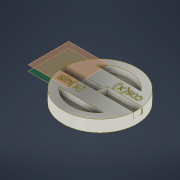
# Autodesk Inventor part: sincos stand
Saved by Autodesk Inventor 2022 (Build 260153000, 153)
## iProperties
Created: 2021-06-07
Part Number: sincos stand
Material: Generic
Document SubType Name: Modeling
Designer: sidsa
Density: 1 g/cm^3
Appearance: Silver
Author: sidsa
## iProperties of the stored document sincos stand_3DPrint.ipt
Created: 2021-06-07
Part Number: sincos stand_3DPrint
Material: Generic
Document SubType Name: Modeling
Designer: sidsa
Density: 1 g/cm^3
Appearance: Default
Author: sidsa
Autodesk Inventor part; units mm, degrees
ref_plane "YZ Plane" through (0, 0, 0) normal (1, 0, 0) x (0, 1, 0)
ref_plane "XZ Plane" through (0, 0, 0) normal (0, 1, 0) x (-1, 0, 0)
ref_plane "XY Plane" through (0, 0, 0) normal (0, 0, 1) x (1, 0, 0)
sketch "Sketch1" plane through (0, 0, 0) normal (0, 1, 0) x (-1, 0, 0)
  line L0 (0, 0) -> (0, 4.7625) construction
  line L1 (-39.8982, 4.7625) -> (0, 4.7625) construction
  line L2 (-39.8982, 0) -> (-39.8982, 4.7625) construction
  line L3 (-39.8982, 0) -> (-19.9491, 0) construction
  line L4 (-19.9491, 0) -> (-19.9491, 3.175) construction
  line L5 (-19.9491, 3.175) -> (-16.0334, 3.175) construction
  line L6 (-19.9491, 0.5949) -> (0, 0.5949) construction
  line L7 (-19.9491, 3.7699) -> (0, 3.7699) construction
  line L8 (-19.9491, 0.5949) -> (-19.9491, 3.7699) construction
  line L9 (-39.8982, 0) -> (-20.8482, 0)
  line L10 (-20.8482, 0) -> (-20.8482, 4.7625)
  line L11 (-20.8482, 4.7625) -> (-39.8982, 4.7625)
  line L12 (-39.8982, 4.7625) -> (-39.8982, 0)
  circle A0 centre (-19.9491, 2.9762) radius 20.0907
  line L13 (0, 4.7625) -> (-19.9491, 4.7625)
  line L14 (-19.9491, 4.7625) -> (-19.9491, 1.5875)
  line L15 (-19.9491, 1.5875) -> (0, 1.5875)
  line L16 (0, 1.5875) -> (0, 4.7625)
  point P0 (-18.8793, 0.5949)
  point P1 (0, 0.5949)
  point P2 (-39.8182, 0)
  point P3 (-39.8982, 0.5949)
  dimension "d1" = 19.05
  dimension "d15" = 3.175
  constraints: 34 end point, 4 parallel, 4 point on line, 2 horizontal, 2 perpendicular, 3 other
  measures "d1" distance of L11.end L10.end
  measures "d15" distance of L13.end L14.end
extrude "Extrusion5" add sketch "Sketch1" along normal blind 3.175 contours L9 L10 L11 L12 A0 picked at (-7.0697, -0.9692)
ref_plane "Work Plane2" through (0, 0, 0) normal (0, -1, 0) x (1, 0, 0)
sketch "Sketch2" plane through (0, 0, 0) normal (0, -1, 0) x (1, 0, 0)
  circle A0 centre (19.9491, 2.9762) radius 20.0907 projected
  circle A1 centre (19.9491, 2.9762) radius 20.0907
  point P0 (0, 0)
  point P1 (39.8982, 0)
  point P2 (39.8199, 0.0117)
  point P3 (40.0398, 2.9762)
  constraints: 1 centre point, 1 coincident, 1 other
extrude "Extrusion2" add sketch "Sketch2" along normal blind 3.175
ref_plane "Work Plane3" through (0, 3.175, 0) normal (0, 1, 0) x (1, 0, 0)
ref_plane "Work Plane1" through (0, 3.175, 0) normal (0, 1, 0) x (1, 0, 0)
sketch "Sketch4" plane through (0, 3.175, 0) normal (0, 1, 0) x (1, 0, 0)
  circle A0 centre (19.9491, -2.9762) radius 20.0907 projected
  circle A1 centre (19.9491, -2.9762) radius 20.0289
  circle A2 centre (19.9491, -2.9762) radius 15.875
  line L0 (32.1471, 7.1838) -> (7.7512, 7.1838)
  line L1 (7.7512, -13.1362) -> (32.1471, -13.1362)
  point P0 (0, 0)
  point P1 (39.8982, -4.7625)
  dimension "d9" = 31.75
  dimension "d10" = 10.16
  dimension "d11" = 10.16
  constraints: 4 end point, 4 point on circle, 2 coincident, 1 centre point, 1 horizontal, 1 parallel, 4 other
  measures "d9" diameter of A2
  measures "d10" distance from line of A2.centre L0
  measures "d11" distance from line of A2.centre L1
extrude "Extrusion4" cut sketch "Sketch4" against normal blind 3.175 contours L0 A2 | A2 L1
sketch "Sketch3" plane through (0, 3.175, 0) normal (0, 1, 0) x (1, 0, 0)
  line L0 (2.8498, -5.5048) -> (33.0797, -5.5048) construction
  line L1 (33.0797, -5.5048) -> (33.0797, -13.0442) construction
  line L2 (33.0797, -13.0442) -> (2.8498, -13.0442) construction
  line L3 (2.8498, -13.0442) -> (2.8498, -5.5048) construction
  line L4 (36.2628, 0.6402) -> (6.0329, 0.6402) construction
  line L5 (6.0329, 0.6402) -> (6.0329, 10.1631) construction
  line L6 (6.0329, 10.1631) -> (36.2628, 10.1631) construction
  line L7 (36.2628, 10.1631) -> (36.2628, 0.6402) construction
  spline S0 degree 2 poles (34.7777, 4.6848) (35.0741, 4.6848) (35.565, 4.5027) (35.741, 4.3174) knots 0 0 0 1 2 2 2
  spline S1 degree 2 poles (35.741, 4.3174) (35.917, 4.1353) (36.1115, 3.5733) (36.1115, 3.1967) knots 0 0 0 1 2 2 2
  spline S2 degree 2 poles (36.1115, 3.1967) (36.1115, 2.82) (35.9108, 2.2704) (35.741, 2.0851) knots 0 0 0 1 2 2 2
  spline S3 degree 2 poles (35.741, 2.0851) (35.5712, 1.8968) (35.0679, 1.6961) (34.7777, 1.6961) knots 0 0 0 1 2 2 2
  spline S4 degree 2 poles (34.7777, 1.6961) (34.543, 1.6961) (34.1046, 1.8289) (33.9348, 1.9153) knots 0 0 0 1 2 2 2
  line L8 (33.9348, 1.9153) -> (33.9348, 2.4556)
  line L9 (33.9348, 2.4556) -> (33.9626, 2.4556)
  spline S5 degree 2 poles (33.9626, 2.4556) (34.0151, 2.4124) (34.1756, 2.3013) (34.2898, 2.2426) knots 0 0 0 1 2 2 2
  spline S6 degree 2 poles (34.2898, 2.2426) (34.3917, 2.1932) (34.6634, 2.116) (34.7869, 2.116) knots 0 0 0 1 2 2 2
  spline S7 degree 2 poles (34.7869, 2.116) (35.1605, 2.116) (35.6144, 2.681) (35.6144, 3.1967) knots 0 0 0 1 2 2 2
  spline S8 degree 2 poles (35.6144, 3.1967) (35.6144, 3.6999) (35.176, 4.2649) (34.7869, 4.2649) knots 0 0 0 1 2 2 2
  spline S9 degree 2 poles (34.7869, 4.2649) (34.5523, 4.2649) (34.1262, 4.0704) (33.9626, 3.9191) knots 0 0 0 1 2 2 2
  line L10 (33.9626, 3.9191) -> (33.9348, 3.9191)
  line L11 (33.9348, 3.9191) -> (33.9348, 4.4594)
  spline S10 degree 2 poles (33.9348, 4.4594) (34.0058, 4.4934) (34.2219, 4.5891) (34.3084, 4.6107) knots 0 0 0 1 2 2 2
  spline S11 degree 2 poles (34.3084, 4.6107) (34.4319, 4.6478) (34.6264, 4.6848) (34.7777, 4.6848) knots 0 0 0 1 2 2 2
  spline S12 degree 2 poles (31.1468, 3.1905) (31.1468, 3.913) (31.8414, 4.7003) (32.4219, 4.7003) knots 0 0 0 1 2 2 2
  spline S13 degree 2 poles (32.4219, 4.7003) (33.0178, 4.7003) (33.7001, 3.8883) (33.7001, 3.1905) knots 0 0 0 1 2 2 2
  spline S14 degree 2 poles (33.7001, 3.1905) (33.7001, 2.4742) (32.9962, 1.6807) (32.4219, 1.6807) knots 0 0 0 1 2 2 2
  spline S15 degree 2 poles (32.4219, 1.6807) (31.8414, 1.6807) (31.1468, 2.4711) (31.1468, 3.1905) knots 0 0 0 1 2 2 2
  spline S16 degree 2 poles (31.6438, 3.1905) (31.6438, 2.6347) (32.0483, 2.0944) (32.4219, 2.0944) knots 0 0 0 1 2 2 2
  spline S17 degree 2 poles (32.4219, 2.0944) (32.7955, 2.0944) (33.203, 2.6347) (33.203, 3.1905) knots 0 0 0 1 2 2 2
  spline S18 degree 2 poles (33.203, 3.1905) (33.203, 3.7308) (32.7955, 4.2865) (32.4219, 4.2865) knots 0 0 0 1 2 2 2
  spline S19 degree 2 poles (32.4219, 4.2865) (32.0514, 4.2865) (31.6438, 3.7401) (31.6438, 3.1905) knots 0 0 0 1 2 2 2
  spline S20 degree 2 poles (29.8809, 4.6879) (30.168, 4.6879) (30.6651, 4.5335) (30.8287, 4.4471) knots 0 0 0 1 2 2 2
  line L12 (30.8287, 4.4471) -> (30.8287, 3.9068)
  line L13 (30.8287, 3.9068) -> (30.804, 3.9068)
  spline S21 degree 2 poles (30.804, 3.9068) (30.7423, 3.9562) (30.5756, 4.0735) (30.4366, 4.1383) knots 0 0 0 1 2 2 2
  spline S22 degree 2 poles (30.4366, 4.1383) (30.3162, 4.197) (30.0198, 4.2835) (29.8623, 4.2835) knots 0 0 0 1 2 2 2
  spline S23 degree 2 poles (29.8623, 4.2835) (29.7481, 4.2835) (29.4857, 4.231) (29.4239, 4.1877) knots 0 0 0 1 2 2 2
  spline S24 degree 2 poles (29.4239, 4.1877) (29.3344, 4.1291) (29.2541, 3.9963) (29.2541, 3.8605) knots 0 0 0 1 2 2 2
  spline S25 degree 2 poles (29.2541, 3.8605) (29.2541, 3.6907) (29.4394, 3.5147) (29.6771, 3.456) knots 0 0 0 1 2 2 2
  spline S26 degree 2 poles (29.6771, 3.456) (29.7697, 3.4344) (30.0661, 3.3726) (30.1927, 3.3387) knots 0 0 0 1 2 2 2
  spline S27 degree 2 poles (30.1927, 3.3387) (30.52, 3.243) (30.8164, 2.8478) (30.8164, 2.5668) knots 0 0 0 1 2 2 2
  spline S28 degree 2 poles (30.8164, 2.5668) (30.8164, 2.1778) (30.2328, 1.693) (29.7512, 1.693) knots 0 0 0 1 2 2 2
  spline S29 degree 2 poles (29.7512, 1.693) (29.5135, 1.693) (29.0318, 1.8104) (28.8682, 1.8999) knots 0 0 0 1 2 2 2
  line L14 (28.8682, 1.8999) -> (28.8682, 2.4155)
  line L15 (28.8682, 2.4155) -> (28.8929, 2.4155)
  spline S30 degree 2 poles (28.8929, 2.4155) (29.0781, 2.2673) (29.5289, 2.0975) (29.7605, 2.0975) knots 0 0 0 1 2 2 2
  spline S31 degree 2 poles (29.7605, 2.0975) (29.9982, 2.0975) (30.3255, 2.2982) (30.3255, 2.4989) knots 0 0 0 1 2 2 2
  spline S32 degree 2 poles (30.3255, 2.4989) (30.3255, 2.681) (30.131, 2.857) (29.9148, 2.9126) knots 0 0 0 1 2 2 2
  spline S33 degree 2 poles (29.9148, 2.9126) (29.8099, 2.9404) (29.5443, 2.996) (29.3992, 3.0299) knots 0 0 0 1 2 2 2
  spline S34 degree 2 poles (29.3992, 3.0299) (29.0843, 3.1102) (28.7632, 3.4776) (28.7632, 3.7956) knots 0 0 0 1 2 2 2
  spline S35 degree 2 poles (28.7632, 3.7956) (28.7632, 3.9809) (28.9083, 4.3082) (29.0503, 4.4286) knots 0 0 0 1 2 2 2
  spline S36 degree 2 poles (29.0503, 4.4286) (29.2016, 4.5552) (29.5876, 4.6879) (29.8809, 4.6879) knots 0 0 0 1 2 2 2
  line L16 (26.8489, 5.6728) -> (27.4356, 5.6728)
  spline S37 degree 2 poles (27.4356, 5.6728) (27.8802, 5.1449) (28.3896, 3.9624) (28.3896, 3.1565) knots 0 0 0 1 2 2 2
  spline S38 degree 2 poles (28.3896, 3.1565) (28.3896, 2.3692) (27.8863, 1.1682) (27.4356, 0.6402) knots 0 0 0 1 2 2 2
  line L17 (27.4356, 0.6402) -> (26.8489, 0.6402)
  line L18 (26.8489, 0.6402) -> (26.8489, 0.6649)
  spline S39 degree 2 poles (26.8489, 0.6649) (27.0558, 0.8532) (27.4325, 1.3411) (27.593, 1.6652) knots 0 0 0 1 2 2 2
  spline S40 degree 2 poles (27.593, 1.6652) (27.7474, 1.9802) (27.9388, 2.7366) (27.9388, 3.1565) knots 0 0 0 1 2 2 2
  spline S41 degree 2 poles (27.9388, 3.1565) (27.9388, 3.5949) (27.7536, 4.3205) (27.593, 4.6478) knots 0 0 0 1 2 2 2
  spline S42 degree 2 poles (27.593, 4.6478) (27.4386, 4.9627) (27.0465, 5.4722) (26.8489, 5.6481) knots 0 0 0 1 2 2 2
  line L19 (26.8489, 5.6481) -> (26.8489, 5.6728)
  line L20 (24.0887, 4.62) -> (24.6784, 4.62)
  line L21 (24.6784, 4.62) -> (25.3731, 3.5455)
  line L22 (25.3731, 3.5455) -> (26.0863, 4.62)
  line L23 (26.0863, 4.62) -> (26.6328, 4.62)
  line L24 (26.6328, 4.62) -> (25.6417, 3.2028)
  line L25 (25.6417, 3.2028) -> (26.6235, 1.761)
  line L26 (26.6235, 1.761) -> (26.0338, 1.761)
  line L27 (26.0338, 1.761) -> (25.3422, 2.8262)
  line L28 (25.3422, 2.8262) -> (24.6352, 1.761)
  line L29 (24.6352, 1.761) -> (24.0887, 1.761)
  line L30 (24.0887, 1.761) -> (25.0736, 3.172)
  line L31 (25.0736, 3.172) -> (24.0887, 4.62)
  spline S43 degree 2 poles (22.3319, 3.1565) (22.3319, 3.9469) (22.8382, 5.1449) (23.2859, 5.6728) knots 0 0 0 1 2 2 2
  line L32 (23.2859, 5.6728) -> (23.8726, 5.6728)
  line L33 (23.8726, 5.6728) -> (23.8726, 5.6481)
  spline S44 degree 2 poles (23.8726, 5.6481) (23.675, 5.4722) (23.2767, 4.9565) (23.1285, 4.6478) knots 0 0 0 1 2 2 2
  spline S45 degree 2 poles (23.1285, 4.6478) (22.9679, 4.3174) (22.7827, 3.5826) (22.7827, 3.1565) knots 0 0 0 1 2 2 2
  spline S46 degree 2 poles (22.7827, 3.1565) (22.7827, 2.7335) (22.971, 1.9833) (23.1285, 1.6652) knots 0 0 0 1 2 2 2
  spline S47 degree 2 poles (23.1285, 1.6652) (23.2828, 1.3472) (23.678, 0.8409) (23.8726, 0.6649) knots 0 0 0 1 2 2 2
  line L34 (23.8726, 0.6649) -> (23.8726, 0.6402)
  line L35 (23.8726, 0.6402) -> (23.2859, 0.6402)
  spline S48 degree 2 poles (23.2859, 0.6402) (22.8413, 1.1682) (22.3319, 2.3599) (22.3319, 3.1565) knots 0 0 0 1 2 2 2
  spline S49 degree 2 poles (3.9706, -9.5525) (3.6835, -9.5525) (3.1864, -9.3982) (3.0227, -9.3117) knots 0 0 0 1 2 2 2
  line L36 (3.0227, -9.3117) -> (3.0227, -8.7714)
  line L37 (3.0227, -8.7714) -> (3.0474, -8.7714)
  spline S50 degree 2 poles (3.0474, -8.7714) (3.1092, -8.8208) (3.2759, -8.9381) (3.4148, -9.003) knots 0 0 0 1 2 2 2
  spline S51 degree 2 poles (3.4148, -9.003) (3.5353, -9.0616) (3.8317, -9.1481) (3.9891, -9.1481) knots 0 0 0 1 2 2 2
  spline S52 degree 2 poles (3.9891, -9.1481) (4.1034, -9.1481) (4.3658, -9.0956) (4.4276, -9.0524) knots 0 0 0 1 2 2 2
  spline S53 degree 2 poles (4.4276, -9.0524) (4.5171, -8.9937) (4.5974, -8.8609) (4.5974, -8.7251) knots 0 0 0 1 2 2 2
  spline S54 degree 2 poles (4.5974, -8.7251) (4.5974, -8.5553) (4.4121, -8.3793) (4.1744, -8.3206) knots 0 0 0 1 2 2 2
  spline S55 degree 2 poles (4.1744, -8.3206) (4.0818, -8.299) (3.7853, -8.2373) (3.6588, -8.2033) knots 0 0 0 1 2 2 2
  spline S56 degree 2 poles (3.6588, -8.2033) (3.3315, -8.1076) (3.0351, -7.7124) (3.0351, -7.4314) knots 0 0 0 1 2 2 2
  spline S57 degree 2 poles (3.0351, -7.4314) (3.0351, -7.0424) (3.6186, -6.5577) (4.1003, -6.5577) knots 0 0 0 1 2 2 2
  spline S58 degree 2 poles (4.1003, -6.5577) (4.338, -6.5577) (4.8197, -6.675) (4.9833, -6.7645) knots 0 0 0 1 2 2 2
  line L38 (4.9833, -6.7645) -> (4.9833, -7.2801)
  line L39 (4.9833, -7.2801) -> (4.9586, -7.2801)
  spline S59 degree 2 poles (4.9586, -7.2801) (4.7734, -7.1319) (4.3226, -6.9621) (4.091, -6.9621) knots 0 0 0 1 2 2 2
  spline S60 degree 2 poles (4.091, -6.9621) (3.8533, -6.9621) (3.526, -7.1628) (3.526, -7.3635) knots 0 0 0 1 2 2 2
  spline S61 degree 2 poles (3.526, -7.3635) (3.526, -7.5457) (3.7205, -7.7216) (3.9366, -7.7772) knots 0 0 0 1 2 2 2
  spline S62 degree 2 poles (3.9366, -7.7772) (4.0416, -7.805) (4.3071, -7.8606) (4.4523, -7.8946) knots 0 0 0 1 2 2 2
  spline S63 degree 2 poles (4.4523, -7.8946) (4.7672, -7.9748) (5.0883, -8.3422) (5.0883, -8.6603) knots 0 0 0 1 2 2 2
  spline S64 degree 2 poles (5.0883, -8.6603) (5.0883, -8.8455) (4.9432, -9.1728) (4.8011, -9.2932) knots 0 0 0 1 2 2 2
  spline S65 degree 2 poles (4.8011, -9.2932) (4.6499, -9.4198) (4.2639, -9.5525) (3.9706, -9.5525) knots 0 0 0 1 2 2 2
  line L40 (6.0269, -9.4846) -> (5.5452, -9.4846)
  line L41 (5.5452, -9.4846) -> (5.5452, -6.6256)
  line L42 (5.5452, -6.6256) -> (6.0269, -6.6256)
  line L43 (6.0269, -6.6256) -> (6.0269, -9.4846)
  line L44 (6.0609, -6.1501) -> (5.5144, -6.1501)
  line L45 (5.5144, -6.1501) -> (5.5144, -5.6499)
  line L46 (5.5144, -5.6499) -> (6.0609, -5.6499)
  line L47 (6.0609, -5.6499) -> (6.0609, -6.1501)
  line L48 (8.9786, -9.4846) -> (8.4969, -9.4846)
  line L49 (8.4969, -9.4846) -> (8.4969, -7.8544)
  spline S66 degree 2 poles (8.4969, -7.8544) (8.4969, -7.6568) (8.4599, -7.3172) (8.4043, -7.2153) knots 0 0 0 1 2 2 2
  spline S67 degree 2 poles (8.4043, -7.2153) (8.3456, -7.1072) (8.1357, -7.0023) (7.9566, -7.0023) knots 0 0 0 1 2 2 2
  spline S68 degree 2 poles (7.9566, -7.0023) (7.7775, -7.0023) (7.3977, -7.1937) (7.2156, -7.3481) knots 0 0 0 1 2 2 2
  line L50 (7.2156, -7.3481) -> (7.2156, -9.4846)
  line L51 (7.2156, -9.4846) -> (6.7339, -9.4846)
  line L52 (6.7339, -9.4846) -> (6.7339, -6.6256)
  line L53 (6.7339, -6.6256) -> (7.2156, -6.6256)
  line L54 (7.2156, -6.6256) -> (7.2156, -6.9436)
  spline S69 degree 2 poles (7.2156, -6.9436) (7.4317, -6.7491) (7.8485, -6.5453) (8.0832, -6.5453) knots 0 0 0 1 2 2 2
  spline S70 degree 2 poles (8.0832, -6.5453) (8.5031, -6.5453) (8.9786, -7.1011) (8.9786, -7.629) knots 0 0 0 1 2 2 2
  line L55 (8.9786, -7.629) -> (8.9786, -9.4846)
  line L56 (11.1213, -10.5375) -> (10.5347, -10.5375)
  spline S71 degree 2 poles (10.5347, -10.5375) (10.0901, -10.0095) (9.5806, -8.827) (9.5806, -8.0211) knots 0 0 0 1 2 2 2
  spline S72 degree 2 poles (9.5806, -8.0211) (9.5806, -7.2338) (10.0839, -6.0328) (10.5347, -5.5048) knots 0 0 0 1 2 2 2
  line L57 (10.5347, -5.5048) -> (11.1213, -5.5048)
  line L58 (11.1213, -5.5048) -> (11.1213, -5.5295)
  spline S73 degree 2 poles (11.1213, -5.5295) (10.9144, -5.7178) (10.5378, -6.2057) (10.3772, -6.5299) knots 0 0 0 1 2 2 2
  spline S74 degree 2 poles (10.3772, -6.5299) (10.2228, -6.8448) (10.0314, -7.6012) (10.0314, -8.0211) knots 0 0 0 1 2 2 2
  spline S75 degree 2 poles (10.0314, -8.0211) (10.0314, -8.4596) (10.2167, -9.1851) (10.3772, -9.5124) knots 0 0 0 1 2 2 2
  spline S76 degree 2 poles (10.3772, -9.5124) (10.5316, -9.8273) (10.9237, -10.3368) (11.1213, -10.5128) knots 0 0 0 1 2 2 2
  line L59 (11.1213, -10.5128) -> (11.1213, -10.5375)
  line L60 (13.8815, -9.4846) -> (13.2918, -9.4846)
  line L61 (13.2918, -9.4846) -> (12.5971, -8.4102)
  line L62 (12.5971, -8.4102) -> (11.8839, -9.4846)
  line L63 (11.8839, -9.4846) -> (11.3374, -9.4846)
  line L64 (11.3374, -9.4846) -> (12.3285, -8.0675)
  line L65 (12.3285, -8.0675) -> (11.3467, -6.6256)
  line L66 (11.3467, -6.6256) -> (11.9364, -6.6256)
  line L67 (11.9364, -6.6256) -> (12.628, -7.6908)
  line L68 (12.628, -7.6908) -> (13.335, -6.6256)
  line L69 (13.335, -6.6256) -> (13.8815, -6.6256)
  line L70 (13.8815, -6.6256) -> (12.8966, -8.0366)
  line L71 (12.8966, -8.0366) -> (13.8815, -9.4846)
  spline S77 degree 2 poles (15.6383, -8.0211) (15.6383, -8.8115) (15.132, -10.0095) (14.6843, -10.5375) knots 0 0 0 1 2 2 2
  line L72 (14.6843, -10.5375) -> (14.0977, -10.5375)
  line L73 (14.0977, -10.5375) -> (14.0977, -10.5128)
  spline S78 degree 2 poles (14.0977, -10.5128) (14.2953, -10.3368) (14.6936, -9.8212) (14.8418, -9.5124) knots 0 0 0 1 2 2 2
  spline S79 degree 2 poles (14.8418, -9.5124) (15.0023, -9.182) (15.1876, -8.4472) (15.1876, -8.0211) knots 0 0 0 1 2 2 2
  spline S80 degree 2 poles (15.1876, -8.0211) (15.1876, -7.5981) (14.9992, -6.8479) (14.8418, -6.5299) knots 0 0 0 1 2 2 2
  spline S81 degree 2 poles (14.8418, -6.5299) (14.6874, -6.2119) (14.2922, -5.7055) (14.0977, -5.5295) knots 0 0 0 1 2 2 2
  line L74 (14.0977, -5.5295) -> (14.0977, -5.5048)
  line L75 (14.0977, -5.5048) -> (14.6843, -5.5048)
  spline S82 degree 2 poles (14.6843, -5.5048) (15.1289, -6.0328) (15.6383, -7.2246) (15.6383, -8.0211) knots 0 0 0 1 2 2 2
  point P0 (0, 0)
  constraints: 4 other
extrude "Extrusion3" cut sketch "Sketch3" against normal blind 0.7937
body "Solid1"
